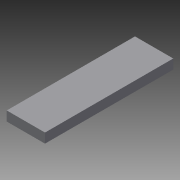
# Autodesk Inventor part: Spacer
Saved by Autodesk Inventor 2013 (Build 170138000, 138)
## iProperties
Created: 2014-02-04
Part Number: Spacer
Material: Generic
Document SubType Name: Modeling
Designer: sethbattis
Density: 1 g/cm^3
Author: sethbattis
Autodesk Inventor part; units mm, degrees
ref_plane "YZ Plane" through (0, 0, 0) normal (1, 0, 0) x (0, 1, 0)
ref_plane "XZ Plane" through (0, 0, 0) normal (0, 1, 0) x (-1, 0, 0)
ref_plane "XY Plane" through (0, 0, 0) normal (0, 0, 1) x (1, 0, 0)
sketch "Sketch1" plane through (0, 0, 0) normal (0, 1, 0) x (-1, 0, 0)
  line L0 (-9.7861, 13.5247) -> (15.6139, 13.5247)
  line L1 (15.6139, 13.5247) -> (15.6139, -71.5653)
  line L2 (15.6139, -71.5653) -> (-9.7861, -71.5653)
  line L3 (-9.7861, -71.5653) -> (-9.7861, 13.5247)
  point P0 (0, 0)
  dimension "d0" = 25.4
  dimension "d2" = 85.09
  constraints: 8 end point, 2 parallel, 1 horizontal, 1 perpendicular
  measures "d0" distance of L0.start L0.end
  measures "d2" distance of L0.end L1.end
extrude "Extrusion1" add sketch "Sketch1" along normal blind 6.35
body "Solid1"
